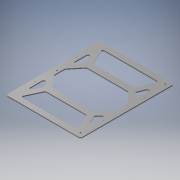
# Autodesk Inventor part: ZBedPlate
Saved by Autodesk Inventor 2016 (Build 200138000, 138)
## iProperties
Category: Sheet Metal
Created: 2015-01-11
Part Number: ZBedPlate
Material: Steel, Alloy
Document SubType Name: Modeling
Designer: Jack
Density: 7.73 g/cm^3
Appearance: Semi-Polished
Mass: 734.813 g
Surface Area: 727.52 cm^2
Volume: 95.0599 cm^3
Author: Jack
Title: Bed Support Plate
Autodesk Inventor part; units mm, degrees
ref_plane "YZ Plane" through (0, 0, 0) normal (1, 0, 0) x (0, 1, 0)
ref_plane "XZ Plane" through (0, 0, 0) normal (0, 1, 0) x (-1, 0, 0)
ref_plane "XY Plane" through (0, 0, 0) normal (0, 0, 1) x (1, 0, 0)
sketch "Sketch1" plane through (0, 0, 0) normal (0, 0, 1) x (1, 0, 0)
  line L0 (0, 0) -> (236.5, 0)
  line L1 (236.5, 0) -> (236.5, 296)
  line L2 (236.5, 296) -> (0, 296)
  line L3 (0, 296) -> (0, 0)
  dimension "d0" = 236.5
  dimension "d1" = 296
  constraints: 8 end point, 2 parallel, 1 horizontal, 1 perpendicular
  measures "d0" distance of L0.start L0.end
  measures "d1" distance of L2.end L0.start
extrude "Extrusion1" add sketch "Sketch1" along normal blind 3
sketch "Sketch2" plane through (0, 0, 3) normal (0, 0, 1) x (1, 0, 0)
  line L0 (0, 0) -> (236.5, 0) projected
  line L1 (236.5, 0) -> (236.5, 296) projected
  line L2 (236.5, 296) -> (0, 296) projected
  line L3 (0, 296) -> (0, 0) projected
  line L4 (206.73, 278) -> (26.73, 278)
  line L5 (26.73, 278) -> (52.377, 223)
  line L6 (52.377, 223) -> (183.9694, 223)
  line L7 (183.9694, 223) -> (206.73, 278)
  line L8 (216.5, 259.7655) -> (196.986, 212.6108)
  line L9 (196.986, 212.6108) -> (216.5, 193.0968)
  line L10 (218.5, 168.4694) -> (183.9694, 203)
  line L11 (216.5, 259.7655) -> (216.5, 193.0968)
  line L12 (183.9694, 203) -> (52.377, 203)
  line L13 (52.377, 203) -> (21.4564, 165.2026)
  line L14 (18, 258.8624) -> (39.5675, 212.6108)
  line L15 (39.5675, 212.6108) -> (18, 186.2467)
  line L16 (18, 186.2467) -> (18, 258.8624)
  line L17 (21.4564, 130.7974) -> (52.377, 93)
  line L18 (52.377, 93) -> (183.9694, 93)
  line L19 (183.9694, 93) -> (218.5, 127.5306)
  line L20 (218.5, 127.5306) -> (218.5, 168.4694)
  line L21 (216.5, 102.9032) -> (196.986, 83.3892)
  line L22 (196.986, 83.3892) -> (216.5, 36.2345)
  line L23 (216.5, 36.2345) -> (216.5, 102.9032)
  line L24 (18, 109.7533) -> (39.5675, 83.3892)
  line L25 (39.5675, 83.3892) -> (18, 37.1376)
  line L26 (18, 37.1376) -> (18, 109.7533)
  line L27 (26.73, 18) -> (206.73, 18)
  line L28 (206.73, 18) -> (183.9694, 73)
  line L29 (183.9694, 73) -> (52.377, 73)
  line L30 (52.377, 73) -> (26.73, 18)
  line L31 (21.4564, 130.7974) -> (21.4564, 165.2026)
  dimension "d19" = 65
  dimension "d29" = 110
  dimension "d31" = 20
  dimension "d32" = 18
  dimension "d33" = 18
  dimension "d34" = 20
  dimension "d35" = 18
  dimension "d40" = 16
  dimension "d41" = 16
  dimension "d52" = 180
  dimension "d55" = 135
  dimension "d59" = 20
  dimension "d60" = 16
  dimension "d61" = 16
  dimension "d62" = 16
  dimension "d63" = 16
  dimension "d64" = 18
  constraints: 56 end point, 11 parallel, 9 vertical alignment, 8 equal length, 5 vertical, 4 horizontal, 2 horizontal alignment
  measures "d19" angle of L27 L30
  measures "d29" distance between parallel lines of L18 L12
  measures "d31" distance between parallel lines of L6 L12
  measures "d32" distance between parallel lines of L2 L4
  measures "d33" distance between parallel lines of L0 L27
  measures "d34" distance between parallel lines of L1 L11
  measures "d35" distance between parallel lines of L3 L16
  measures "d40" distance between parallel lines of L13 L15
  measures "d41" distance between parallel lines of L9 L10
  measures "d52" distance of L27.start L27.end
  measures "d55" angle of L12 L10
  measures "d59" distance between parallel lines of L29 L18
  measures "d60" distance between parallel lines of L30 L25
  measures "d61" distance between parallel lines of L22 L28
  measures "d62" distance between parallel lines of L8 L7
  measures "d63" distance between parallel lines of L14 L5
  measures "d64" distance between parallel lines of L1 L20
extrude "Extrusion2" cut sketch "Sketch2" against normal up to next contours L7 L6 L5 L4 | L11 L9 L8 | L20 L19 L18 L17 L31 L13 L12 L10 | L14 L15 L16 | L23 L22 L21 | L24 L25 L26 | L30 L29 L28 L27
sketch "Sketch3" plane through (0, 0, 3) normal (0, 0, 1) x (1, 0, 0)
  line L0 (0, 0) -> (236.5, 0) projected
  line L1 (236.5, 0) -> (236.5, 296) projected
  line L2 (236.5, 296) -> (0, 296) projected
  line L3 (0, 296) -> (0, 0) projected
  circle A0 centre (222.5, 282) radius 2.25
  circle A1 centre (14, 148) radius 2.25
  circle A2 centre (222.5, 14) radius 2.25
  dimension "d44" = 4.5
  dimension "d45" = 14
  dimension "d46" = 14
  dimension "d47" = 14
  dimension "d56" = 148
  dimension "d57" = 14
  constraints: 3 centre point, 2 equal radius, 1 vertical alignment
  measures "d44" diameter of A0
  measures "d45" distance from line of L1 A0.centre
  measures "d46" distance from line of L2 A0.centre
  measures "d47" distance from line of L0 A2.centre
  measures "d56" distance from line of L2 A1.centre
  measures "d57" distance from line of L3 A1.centre
extrude "Extrusion3" cut sketch "Sketch3" against normal up to next contours A0 | A1 | A2
fillet "Fillet1" radius 4.7625 28 edges at (26.73, 18, 1.5) (206.73, 18, 1.5) (183.9694, 73, 1.5) (52.377, 73, 1.5) (18, 37.1376, 1.5) (39.5675, 83.3892, 1.5) (18, 109.7533, 1.5) (39.5675, 212.6108, 1.5) (18, 186.2467, 1.5) (18, 258.8624, 1.5) (26.73, 278, 1.5) (52.377, 223, 1.5) (183.9694, 223, 1.5) (206.73, 278, 1.5) (196.986, 83.3892, 1.5) (216.5, 36.2345, 1.5) (216.5, 102.9032, 1.5) (216.5, 193.0968, 1.5) (196.986, 212.6108, 1.5) (216.5, 259.7655, 1.5) (218.5, 127.5306, 1.5) (218.5, 168.4694, 1.5) (183.9694, 93, 1.5) (183.9694, 203, 1.5) (52.377, 203, 1.5) (21.4564, 165.2026, 1.5) (21.4564, 130.7974, 1.5) (52.377, 93, 1.5)
fillet "Fillet2" radius 5 4 edges at (236.5, 0, 1.5) (0, 0, 1.5) (0, 296, 1.5) (236.5, 296, 1.5)
sketch "Sketch4" plane through (0, 0, 0) normal (0, 0, -1) x (-1, 0, 0)
  line L0 (-181.9967, 203) -> (-54.634, 203) projected
  line L1 (-54.634, 93) -> (-181.9967, 93) projected
  line L2 (-236.5, 5) -> (-236.5, 291) projected
  line L3 (0, 291) -> (0, 5) projected
  point P0 (0, 0)
  point P1 (-10, 213)
  point P2 (-226.5, 213)
  point P3 (-10, 83)
  point P4 (-226.5, 83)
  dimension "d65" = 10
  dimension "d66" = 10
  dimension "d67" = 10
  dimension "d68" = 10
  constraints: 2 horizontal alignment, 2 vertical alignment
  measures "d65" distance from line of point (-10, 213) L0
  measures "d66" distance from line of point (-10, 83) L1
  measures "d67" distance from line of L2 point (-226.5, 83)
  measures "d68" distance from line of L3 point (-10, 83)
hole "Hole1" at (10, 213, 0) at (226.5, 213, 0) at (10, 83, 0) at (226.5, 83, 0) direction (0, 0, 1) diameter 4 end through all countersink diameter 8 countersink angle 90
body "Solid1"
